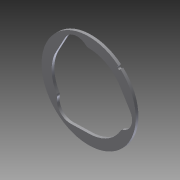
# Autodesk Inventor part: launcher.cam
Saved by Autodesk Inventor 2011 (Build 150239000, 239)
## iProperties
Created: 2011-02-22
Part Number: launcher.cam
Document SubType Name: Modeling
Designer: Casey
Density: 1 g/cm^3
Mass: 19.7834 g
Surface Area: 131.71 cm^2
Volume: 19.7834 cm^3
Author: Casey
Autodesk Inventor part; units mm, degrees
ref_plane "YZ Plane" through (0, 0, 0) normal (1, 0, 0) x (0, 1, 0)
ref_plane "XZ Plane" through (0, 0, 0) normal (0, 1, 0) x (-1, 0, 0)
ref_plane "XY Plane" through (0, 0, 0) normal (0, 0, 1) x (1, 0, 0)
sketch "Sketch2" plane through (0, 0, 0) normal (0, 1, 0) x (-1, 0, 0)
  circle A0 centre (0, 0) radius 55
  circle A1 centre (0, 0) radius 70
  dimension "d18" = 110
  dimension "d19" = 140
  constraints: 2 centre point, 2 coincident
  measures "d18" diameter of A0
  measures "d19" diameter of A1
extrude "Extrusion3" add sketch "Sketch2" along normal blind 4
sketch "Sketch3" plane through (0, 4, 0) normal (0, 1, 0) x (1, 0, 0)
  circle A0 centre (0, 0) radius 55 projected
  circle A1 centre (0, 0) radius 70 projected
  arc A2 (0, -55) -> (-3.9836, -56.5132) centre (0, -61) ccw
  line L0 (0, -70) -> (0, 0) construction
  line L1 (0, 0) -> (-47.6314, -27.5) construction
  circle A3 centre (0, 0) radius 65 construction
  arc A4 (-34.8476, -51.084) -> (-3.9836, -56.5132) centre (-17.2622, -41.5574) ccw
  line L2 (-34.8476, -51.084) -> (-47.3798, -27.9505)
  arc A5 (-47.3798, -27.9505) -> (-47.6411, -27.4832) centre (-64.9651, -37.4771) ccw
  dimension "d24" = 60
  dimension "d31" = 6
  dimension "d33" = 20
  dimension "d34" = 130
  constraints: 9 point on circle, 6 end point, 6 tangent, 4 centre point, 1 coincident, 1 equal radius, 1 point on line, 1 vertical, 1 vertical alignment, 1 other
  measures "d24" angle of L0 L1
  measures "d31" radius of A2
  measures "d33" radius of A4
  measures "d34" diameter of A3
extrude "Extrusion4" cut sketch "Sketch3" against normal blind 6 contours A0 A2 A4 L2 A5
pattern_circular "Circular Pattern2" count 3 over 360 about axis through (0, 0, 0) along (0, 1, 0) of "Extrusion4"
sketch "Sketch4" plane through (0, 0, 0) normal (0, -1, 0) x (1, 0, 0)
  circle A0 centre (45.0297, 52.0628) radius 2.3813 projected
  circle A1 centre (45.0297, 52.0628) radius 2.3813
  constraints: 1 centre point, 1 coincident, 1 concentric
extrude "Extrusion5" cut sketch "Sketch4" against normal blind 5.25
body "Solid3"
